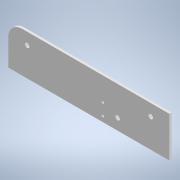
# Autodesk Inventor part: new side of drivetrain
Saved by Autodesk Inventor 2020 (Build 240168000, 168)
## iProperties
Created: 2020-02-25
Part Number: new side of drivetrain
Material: Generic
Document SubType Name: Modeling
Designer: jackm
Density: 1 g/cm^3
Appearance: Default
Author: jackm
Autodesk Inventor part; units mm, degrees
ref_plane "YZ Plane" through (0, 0, 0) normal (1, 0, 0) x (0, 1, 0)
ref_plane "XZ Plane" through (0, 0, 0) normal (0, 1, 0) x (-1, 0, 0)
ref_plane "XY Plane" through (0, 0, 0) normal (0, 0, 1) x (1, 0, 0)
ref_plane "Work Plane1" through (0, 0, 0) normal (0, 0, 1) x (1, 0, 0)
sketch "Sketch1" plane through (0, 0, 0) normal (0, 0, 1) x (1, 0, 0)
  circle A0 centre (258.0538, 71.9271) radius 7 construction
  circle A1 centre (-78.0149, 71.9271) radius 7 construction
  circle A2 centre (258.0538, 71.9271) radius 6.2357
  circle A3 centre (-78.0149, 71.9271) radius 6.2357
  line L0 (258.0538, 71.9271) -> (-78.0149, 71.9271) construction
  line L1 (258.0538, 71.9271) -> (258.0538, 103.6771) construction
  line L2 (-78.0149, 71.9271) -> (-78.0149, 103.6771) construction
  line L3 (258.0538, 103.6771) -> (-78.0149, 103.6771)
  line L4 (-78.0149, 103.6771) -> (-90.9562, 103.6771)
  line L5 (258.0538, 103.6771) -> (309.0951, 103.6771)
  line L6 (0, 0) -> (192, 0) construction
  line L7 (192, 0) -> (192, -6.35) construction
  line L8 (192, -6.35) -> (309.0951, -6.35)
  line L9 (309.0951, -6.35) -> (309.0951, 103.6771)
  line L10 (192, -6.35) -> (-129.0562, -6.35)
  line L11 (-129.0562, -6.35) -> (-129.0562, 65.5771)
  arc A4 (-90.9562, 103.6771) -> (-129.0562, 65.5771) centre (-90.9562, 65.5771) ccw
  arc A5 (164.9838, 25.75) -> (164.9838, 22.25) centre (168.0148, 24) ccw construction
  circle A6 centre (168.0148, 24) radius 6.2357
  circle A7 centre (128, 8) radius 2 construction
  circle A8 centre (128, 40) radius 2 construction
  circle A9 centre (128, 8) radius 3.175
  circle A10 centre (128, 40) radius 3.175
  circle A11 centre (24, 72) radius 4.83 construction
  circle A12 centre (24, 72) radius 6.2357
  circle A13 centre (64, 56) radius 2 construction
  circle A14 centre (64, 88) radius 2 construction
  circle A15 centre (64, 56) radius 3.175
  circle A16 centre (64, 88) radius 3.175
  circle A17 centre (8, 8) radius 2 construction
  circle A18 centre (8, 40) radius 2 construction
  circle A19 centre (184, 8) radius 2 construction
  circle A20 centre (184, 40) radius 2 construction
  circle A21 centre (184, 8) radius 1.778
  circle A22 centre (184, 40) radius 1.778
  circle A23 centre (8, 8) radius 1.778
  circle A24 centre (8, 40) radius 1.778
  point P0 (-129.0562, 103.6771)
  dimension "d0" = 12.4714
  dimension "d1" = 12.4714
  dimension "d2" = 31.75
  dimension "d3" = 31.75
  dimension "d4" = 51.0413
  dimension "d5" = 51.0413
  dimension "d6" = 6.35
  dimension "d7" = 38.1
  dimension "d8" = 12.4714
  dimension "d9" = 6.35
  dimension "d10" = 6.35
  dimension "d13" = 12.4714
  dimension "d14" = 6.35
  dimension "d15" = 6.35
  dimension "d16" = 3.556
  dimension "d17" = 3.556
  dimension "d18" = 3.556
  dimension "d19" = 3.556
  constraints: 22 end point, 13 centre point, 12 coincident, 3 point on line, 3 vertical, 2 horizontal, 2 parallel, 2 perpendicular, 2 point on circle, 2 tangent
  measures "d0" diameter of A2
  measures "d1" diameter of A3
  measures "d2" distance of L0.start L1.end
  measures "d3" distance of L0.end L2.end
  measures "d4" distance of L2.end point (-129.056, 103.677)
  measures "d5" distance of L1.end L5.end
  measures "d6" distance of L6.end L7.end
  measures "d7" radius of A4
  measures "d8" diameter of A6
  measures "d9" diameter of A9
  measures "d10" diameter of A10
  measures "d13" diameter of A12
  measures "d14" diameter of A15
  measures "d15" diameter of A16
  measures "d16" diameter of A21
  measures "d17" diameter of A22
  measures "d18" diameter of A23
  measures "d19" diameter of A24
extrude "Extrusion1" add sketch "Sketch1" along normal blind 6.35 contours L5 L9 L8 L10 L11 A4 L4 L3 | A12 | A15 | A16 | A21 | A22 | A23 | A24
body "Solid1"
